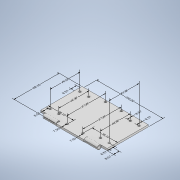
# Autodesk Inventor part: Part3
Saved by Autodesk Inventor 2020 (Build 240168000, 168)
## iProperties
Created: 2019-08-08
Part Number: Part3
Material: Generic
Document SubType Name: Modeling
Designer: Nicolas
Density: 1 g/cm^3
Appearance: Default
Author: Nicolas
Autodesk Inventor part; units mm, degrees
ref_plane "YZ Plane" through (0, 0, 0) normal (1, 0, 0) x (0, 1, 0)
ref_plane "XZ Plane" through (0, 0, 0) normal (0, 1, 0) x (-1, 0, 0)
ref_plane "XY Plane" through (0, 0, 0) normal (0, 0, 1) x (1, 0, 0)
sketch "Sketch1" plane through (0, 0, 0) normal (1, 0, 0) x (0, 1, 0)
  line L0 (3.2531, 52.0584) -> (0.3531, 52.0584)
  line L1 (0.3531, 52.0584) -> (0.3531, -10.0416)
  line L2 (0.3531, -10.0416) -> (3.2531, -10.0416)
  line L3 (3.2531, -10.0416) -> (3.2531, 52.0584)
  arc A0 (3.2531, 52.0584) -> (2.9699, 57.9259) centre (1.8031, 54.929) ccw
  arc A1 (0.7699, 57.9745) -> (0.3531, 52.0584) centre (1.8031, 54.929) ccw
  line L4 (0.7699, 57.9745) -> (0.7699, 56.8745)
  line L5 (2.9699, 57.9259) -> (2.9699, 56.8259)
  arc A2 (0.7699, 56.8745) -> (2.9699, 56.8259) centre (1.8253, 54.832) ccw
  point P0 (0, 0)
  dimension "d0" = 2.9
  dimension "d1" = 62.1
  dimension "d156" = 1.1
  dimension "d157" = 1.1
  dimension "d158" = 2.2
  constraints: 12 end point, 7 point on circle, 3 centre point, 2 parallel, 2 vertical, 1 coincident, 1 horizontal, 1 perpendicular
  measures "d0" distance between parallel lines of L1 L3
  measures "d1" distance between parallel lines of L2 L0
  measures "d156" distance of L5.start L5.end
  measures "d157" distance of L4.start L4.end
  measures "d158" distance between parallel lines of L4 L5
extrude "Extrusion1" add sketch "Sketch1" against normal blind 20
sketch "Sketch3" plane through (0, 0, 0) normal (1, 0, 0) x (0, 0, -1)
  arc A0 (-52.0584, 3.2531) -> (-57.9259, 2.9699) centre (-54.929, 1.8031) ccw projected
  line L0 (10.0416, 0.3531) -> (-52.0584, 0.3531) projected
  line L1 (-52.0584, 3.2531) -> (10.0416, 3.2531)
  line L2 (10.0416, 3.2531) -> (10.0416, 0.3531)
  line L3 (10.0416, 0.3531) -> (-52.0584, 0.3531)
  line L4 (-52.0584, 0.3531) -> (-52.0584, 3.2531)
  point P0 (0, 0)
  constraints: 8 end point, 2 parallel, 1 horizontal, 1 perpendicular
extrude "Extrusion2" add sketch "Sketch3" along normal blind 42.1
sketch "Sketch4" plane through (42.1, 0, 0) normal (1, 0, 0) x (0, 0, -1)
  line L0 (10.0416, 0.3531) -> (-52.0584, 0.3531) projected
  line L1 (10.0416, 0.3531) -> (-52.0584, 0.3531)
  line L2 (-52.0584, 0.3531) -> (-52.0584, 3.2531)
  line L3 (-52.0584, 3.2531) -> (10.0416, 3.2531)
  line L4 (10.0416, 3.2531) -> (10.0416, 0.3531)
  arc A0 (-57.9745, 0.7699) -> (-52.0584, 0.3531) centre (-54.929, 1.8031) ccw projected
  arc A1 (-57.9745, 0.7699) -> (-52.0584, 0.3531) centre (-54.929, 1.8031) ccw
  arc A2 (-52.0584, 3.2531) -> (-57.9259, 2.9699) centre (-54.929, 1.8031) ccw projected
  arc A3 (-52.0584, 3.2531) -> (-57.9259, 2.9699) centre (-54.929, 1.8031) ccw
  arc A4 (-56.8745, 0.7699) -> (-56.8259, 2.9699) centre (-54.832, 1.8253) ccw projected
  arc A5 (-56.8745, 0.7699) -> (-56.8259, 2.9699) centre (-54.832, 1.8253) ccw
  line L5 (-56.8745, 0.7699) -> (-57.9745, 0.7699) projected
  line L6 (-56.8745, 0.7699) -> (-57.9745, 0.7699)
  line L7 (-57.9259, 2.9699) -> (-56.8259, 2.9699) projected
  line L8 (-56.8259, 2.9699) -> (-57.9259, 2.9699)
  point P0 (0, 0)
  dimension "d159" = 1.1
  dimension "d160" = 2.2
  constraints: 12 end point, 6 point on circle, 4 equal length, 3 centre point, 1 coincident, 1 horizontal, 1 perpendicular
  measures "d159" distance of L7.start L7.end
  measures "d160" distance between parallel lines of L5 L7
extrude "Extrusion3" add sketch "Sketch4" along normal blind 20
sketch "Sketch9" plane through (0, 0.3531, 52.0584) normal (0, 0, 1) x (1, 0, 0)
  line L0 (0, 2.9) -> (42.1, 2.9) projected
  line L1 (0, 2.9) -> (42.1, 2.9)
  line L2 (42.1, 2.9) -> (42.1, 0)
  line L3 (42.1, 0) -> (0, 0)
  line L4 (0, 0) -> (0, 2.9)
  point P0 (0, -0.3531)
  constraints: 8 end point, 2 parallel, 1 horizontal, 1 perpendicular
extrude "Extrusion4" add sketch "Sketch9" along normal blind 6
sketch "Sketch10" plane through (-20, 0, 0) normal (-1, 0, 0) x (0, 0, 1)
  arc A0 (52.0584, 0.3531) -> (57.9745, 0.7699) centre (54.929, 1.8031) ccw projected
  line L0 (-10.0416, 3.2531) -> (-10.0416, 0.3531) projected
  line L1 (52.0584, 0.3531) -> (-10.0416, 0.3531)
  line L2 (-10.0416, 0.3531) -> (-10.0416, 3.2531)
  line L3 (-10.0416, 3.2531) -> (52.0584, 3.2531)
  line L4 (52.0584, 3.2531) -> (52.0584, 0.3531)
  point P0 (0, 0)
  constraints: 8 end point, 2 parallel, 1 horizontal, 1 perpendicular
extrude "Extrusion5" add sketch "Sketch10" along normal blind 8.95
sketch "Sketch11" plane through (62.1, 0, 0) normal (1, 0, 0) x (0, 0, -1)
  line L0 (10.0416, 0.3531) -> (10.0416, 3.2531) projected
  arc A0 (-52.0584, 3.2531) -> (-57.7996, 3.2531) centre (-54.929, 1.8031) ccw projected
  line L1 (10.0416, 0.3531) -> (-52.0584, 0.3531)
  line L2 (-52.0584, 0.3531) -> (-52.0584, 3.2531)
  line L3 (-52.0584, 3.2531) -> (10.0416, 3.2531)
  line L4 (10.0416, 3.2531) -> (10.0416, 0.3531)
  point P0 (0, 0)
  constraints: 8 end point, 2 parallel, 1 horizontal, 1 perpendicular
extrude "Extrusion6" add sketch "Sketch11" along normal blind 8.95
sketch "Sketch5" plane through (-20, 0.3531, -10.0416) normal (0, -1, 0) x (1, 0, 0)
  line L0 (20, 62.1) -> (62.1, 62.1) projected
  line L1 (0, 0) -> (0, 62.1) projected
  line L2 (62.1, 68.1) -> (20, 68.1) projected
  line L3 (-8.95, 0) -> (-8.95, 62.1) projected
  point P0 (20, 10.0416)
  point P1 (29.15, 60.6)
  dimension "d80" = 38.1
  dimension "d81" = 7.5
  measures "d80" distance from line of L3 point (29.15, 60.6)
  measures "d81" distance from line of L2 point (29.15, 60.6)
hole "Hole1" at (9.15, 0.3531, 50.5584) direction (0, 1, 0) diameter 2.921 end through all
sketch "Sketch6" plane through (-20, 0.3531, -10.0416) normal (0, -1, 0) x (1, 0, 0)
  line L0 (20, 62.1) -> (62.1, 62.1) projected
  circle A0 centre (29.15, 60.6) radius 1.4605 projected
  line L1 (62.1, 68.1) -> (20, 68.1) projected
  point P0 (20, 10.0416)
  point P1 (52.95, 60.6)
  dimension "d42" = 23.8
  dimension "d53" = 7.5
  measures "d42" distance of point (52.95, 60.6) A0.centre
  measures "d53" distance from line of L1 point (52.95, 60.6)
hole "Hole2" at (32.95, 0.3531, 50.5584) direction (0, 1, 0) diameter 2.921 end through all
sketch "Sketch7" plane through (-20, 0.3531, -10.0416) normal (0, -1, 0) x (1, 0, 0)
  line L0 (0, 0) -> (0, 62.1) projected
  circle A0 centre (29.15, 60.6) radius 1.4605 projected
  line L1 (-8.95, 0) -> (-8.95, 62.1) projected
  point P0 (20, 10.0416)
  point P1 (29.15, 2.71)
  dimension "d49" = 57.89
  dimension "d82" = 38.1
  measures "d49" distance of A0.centre point (29.15, 2.71)
  measures "d82" distance from line of L1 point (29.15, 2.71)
hole "Hole3" at (9.15, 0.3531, -7.3316) direction (0, 1, 0) diameter 2.921 end through all
sketch "Sketch8" plane through (-20, 0.3531, -10.0416) normal (0, -1, 0) x (1, 0, 0)
  circle A0 centre (29.15, 2.71) radius 1.4605 projected
  circle A1 centre (52.95, 60.6) radius 1.4605 projected
  point P0 (20, 10.0416)
  point P1 (52.95, 2.71)
  point P2 (41.1972, 0)
  point P3 (38.7028, 0)
  point P4 (60, 64.989)
  point P5 (60, 63.311)
  dimension "d48" = 23.8
  dimension "d54" = 57.89
  constraints: 2 other
  measures "d48" distance of point (52.95, 2.71) point (29.15, 2.71)
  measures "d54" distance of point (52.95, 60.6) point (52.95, 2.71)
hole "Hole4" at (32.95, 0.3531, -7.3316) direction (0, 1, 0) diameter 2.921 end through all
sketch "Sketch12" plane through (0, 0.3531, 58.0584) normal (0, -1, 0) x (1, 0, 0)
  line L0 (-20, -6) -> (-28.95, -6) projected
  line L1 (-28.95, -68.1) -> (-28.95, -6) projected
  point P0 (0, -58.0584)
  point P1 (-23.54, -14.57)
  dimension "d133" = 8.57
  dimension "d134" = 5.41
  measures "d133" distance from line of L0 point (-23.54, -14.57)
  measures "d134" distance from line of L1 point (-23.54, -14.57)
hole "Hole5" at (-23.54, 0.3531, 43.4884) direction (0, 1, 0) diameter 2.921 end through all
sketch "Sketch13" plane through (0, 0.3531, 58.0584) normal (0, -1, 0) x (1, 0, 0)
  line L0 (0, -6) -> (-20, -6) projected
  circle A0 centre (-23.54, -14.57) radius 1.4605 projected
  point P0 (0, -58.0584)
  point P1 (-10.28, -14.57)
  dimension "d135" = 8.57
  dimension "d136" = 13.26
  measures "d135" distance from line of L0 point (-10.28, -14.57)
  measures "d136" distance of point (-10.28, -14.57) A0.centre
hole "Hole6" at (-10.28, 0.3531, 43.4884) direction (0, 1, 0) diameter 2.921 end through all
sketch "Sketch14" plane through (0, 0.3531, 58.0584) normal (0, -1, 0) x (1, 0, 0)
  line L0 (-28.95, -68.1) -> (-28.95, -6) projected
  circle A0 centre (-23.54, -14.57) radius 1.4605 projected
  point P0 (0, -58.0584)
  point P1 (-23.54, -59.53)
  dimension "d137" = 5.41
  dimension "d138" = 44.96
  measures "d137" distance from line of L0 point (-23.54, -59.53)
  measures "d138" distance of point (-23.54, -59.53) A0.centre
hole "Hole7" at (-23.54, 0.3531, -1.4716) direction (0, 1, 0) diameter 2.921 end through all
sketch "Sketch15" plane through (0, 0.3531, 58.0584) normal (0, -1, 0) x (1, 0, 0)
  circle A0 centre (-10.28, -14.57) radius 1.4605 projected
  circle A1 centre (-23.54, -59.53) radius 1.4605 projected
  point P0 (0, -58.0584)
  point P1 (-10.28, -59.53)
  dimension "d139" = 44.96
  dimension "d148" = 13.26
  measures "d139" distance of A0.centre point (-10.28, -59.53)
  measures "d148" distance of point (-10.28, -59.53) A1.centre
hole "Hole8" at (-10.28, 0.3531, -1.4716) direction (0, 1, 0) diameter 2.921 end through all
sketch "Sketch17" plane through (0, 0.3531, 58.0584) normal (0, -1, 0) x (1, 0, 0)
  line L0 (71.05, -6) -> (71.05, -68.1) projected
  line L1 (62.1, -6) -> (71.05, -6) projected
  point P0 (0, -58.0584)
  point P1 (65.64, -14.57)
  dimension "d142" = 5.41
  dimension "d147" = 8.57
  measures "d142" distance from line of L0 point (65.64, -14.57)
  measures "d147" distance from line of L1 point (65.64, -14.57)
hole "Hole10" at (65.64, 0.3531, 43.4884) direction (0, 1, 0) diameter 2.921 end through all
sketch "Sketch16" plane through (0, 0.3531, 58.0584) normal (0, -1, 0) x (1, 0, 0)
  circle A0 centre (65.64, -14.57) radius 1.4605 projected
  line L0 (42.1, -6) -> (62.1, -6) projected
  point P0 (0, -58.0584)
  point P1 (52.38, -14.57)
  dimension "d144" = 13.26
  dimension "d146" = 8.57
  measures "d144" distance of A0.centre point (52.38, -14.57)
  measures "d146" distance from line of L0 point (52.38, -14.57)
hole "Hole9" at (52.38, 0.3531, 43.4884) direction (0, 1, 0) diameter 2.921 end through all
sketch "Sketch19" plane through (0, 0.3531, 58.0584) normal (0, -1, 0) x (1, 0, 0)
  circle A0 centre (65.64, -14.57) radius 1.4605 projected
  line L0 (71.05, -6) -> (71.05, -68.1) projected
  point P0 (0, -58.0584)
  point P1 (65.64, -59.53)
  dimension "d141" = 44.96
  dimension "d143" = 5.41
  measures "d141" distance of A0.centre point (65.64, -59.53)
  measures "d143" distance from line of L0 point (65.64, -59.53)
hole "Hole12" at (65.64, 0.3531, -1.4716) direction (0, 1, 0) diameter 2.921 end through all
sketch "Sketch18" plane through (0, 0.3531, 58.0584) normal (0, -1, 0) x (1, 0, 0)
  circle A0 centre (52.38, -14.57) radius 1.4605 projected
  circle A1 centre (65.64, -59.53) radius 1.4605 projected
  point P0 (0, -58.0584)
  point P1 (52.38, -59.53)
  dimension "d140" = 44.96
  dimension "d145" = 13.26
  measures "d140" distance of point (52.38, -59.53) A0.centre
  measures "d145" distance of A1.centre point (52.38, -59.53)
hole "Hole11" at (52.38, 0.3531, -1.4716) direction (0, 1, 0) diameter 2.921 end through all
body "Solid1"
